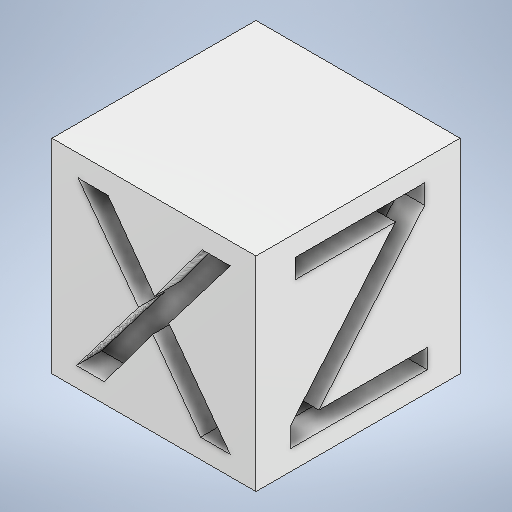
# Autodesk Inventor part: Cubo
Saved by Autodesk Inventor 2025.2 (Build 292293000, 293)
## iProperties
Created: 2025-01-18
Part Number: Cubo
Material: ABS Plastic
Document SubType Name: Modeling
Designer: Tony Dias
Density: 1.06 g/cm^3
Appearance: Smooth - White
Author: Tony Dias
## iProperties of the stored document Cubo_3DPrint.ipt
Created: 2025-01-18
Part Number: Cubo_3DPrint
Material: Generic
Document SubType Name: Modeling
Designer: Tony Dias
Density: 1 g/cm^3
Appearance: Default
Author: Tony Dias
Autodesk Inventor part; units mm, degrees
ref_plane "YZ Plane" through (0, 0, 0) normal (1, 0, 0) x (0, 1, 0)
ref_plane "XZ Plane" through (0, 0, 0) normal (0, 1, 0) x (-1, 0, 0)
ref_plane "XY Plane" through (0, 0, 0) normal (0, 0, 1) x (1, 0, 0)
sketch "Sketch3" plane through (0, 0, 0) normal (0, 0, 1) x (1, 0, 0)
  line L0 (12.7, -12.7) -> (-12.7, -12.7)
  line L1 (-12.7, -12.7) -> (-12.7, 12.7)
  line L2 (-12.7, 12.7) -> (12.7, 12.7)
  line L3 (12.7, 12.7) -> (12.7, -12.7)
  line L4 (12.7, -12.7) -> (-12.7, 12.7) construction
  line L5 (-12.7, -12.7) -> (12.7, 12.7) construction
  point P0 (0, 0)
  dimension "d0" = 25.4
  dimension "d1" = 25.4
  constraints: 12 end point, 2 midpoint, 2 parallel, 1 horizontal, 1 perpendicular
  measures "d0" distance of L1.end L2.end
  measures "d1" distance of L0.end L1.end
extrude "Cubo" add sketch "Sketch3" along normal blind 25.4
sketch "Sketch5" plane through (0, 0, 25.4) normal (0, 0, 1) x (1, 0, 0)
  line L0 (-12.1868, 12.0555) -> (12.0292, 12.0555) construction
  line L1 (12.0292, 12.0555) -> (12.0292, -12.3181) construction
  line L2 (12.0292, -12.3181) -> (-12.1868, -12.3181) construction
  line L3 (-12.1868, -12.3181) -> (-12.1868, 12.0555) construction
  line L4 (9.4966, -10.2913) -> (5.7916, -10.2913)
  line L5 (5.7916, -10.2913) -> (-0.1365, -2.1567)
  line L6 (-0.1365, -2.1567) -> (-6.1633, -10.2913)
  line L7 (-6.1633, -10.2913) -> (-9.6707, -10.2913)
  line L8 (-9.6707, -10.2913) -> (-1.9149, -0.1313)
  line L9 (-1.9149, -0.1313) -> (-9.4402, 10.0287)
  line L10 (-9.4402, 10.0287) -> (-5.7352, 10.0287)
  line L11 (-5.7352, 10.0287) -> (0.0776, 2.0588)
  line L12 (0.0776, 2.0588) -> (5.9892, 10.0287)
  line L13 (5.9892, 10.0287) -> (9.4966, 10.0287)
  line L14 (9.4966, 10.0287) -> (1.856, 0.0169)
  line L15 (1.856, 0.0169) -> (9.4966, -10.2913)
  point P0 (0, 0)
  constraints: 2 other
extrude "X" cut sketch "Sketch5" against normal blind 3.175
sketch "Sketch6" plane through (12.7, -12.7, 0) normal (1, 0, 0) x (0, 0, -1)
  line L0 (-25.0445, 24.9615) -> (-0.3507, 24.9615) construction
  line L1 (-0.3507, 24.9615) -> (-0.3507, 0.3203) construction
  line L2 (-0.3507, 0.3203) -> (-25.0445, 0.3203) construction
  line L3 (-25.0445, 0.3203) -> (-25.0445, 24.9615) construction
  line L4 (-4.069, 2.4809) -> (-21.0792, 2.4809)
  line L5 (-21.0792, 2.4809) -> (-21.0792, 5.0003)
  line L6 (-21.0792, 5.0003) -> (-8.0375, 20.3967)
  line L7 (-8.0375, 20.3967) -> (-20.4864, 20.3967)
  line L8 (-20.4864, 20.3967) -> (-20.4864, 22.8009)
  line L9 (-20.4864, 22.8009) -> (-4.3984, 22.8009)
  line L10 (-4.3984, 22.8009) -> (-4.3984, 20.3638)
  line L11 (-4.3984, 20.3638) -> (-17.5718, 4.885)
  line L12 (-17.5718, 4.885) -> (-4.069, 4.885)
  line L13 (-4.069, 4.885) -> (-4.069, 2.4809)
  point P0 (0, 12.7)
  constraints: 2 other
extrude "Z" cut sketch "Sketch6" against normal blind 3.175
sketch "Sketch7" plane through (0, 0, 0) normal (0, 0, -1) x (-1, 0, 0)
  line L0 (-12.3672, 12.2796) -> (12.4407, 12.2796) construction
  line L1 (12.4407, 12.2796) -> (12.4407, -12.4691) construction
  line L2 (12.4407, -12.4691) -> (-12.3672, -12.4691) construction
  line L3 (-12.3672, -12.4691) -> (-12.3672, 12.2796) construction
  line L4 (-1.8683, -10.2547) -> (-1.8683, -1.7055)
  line L5 (-1.8683, -1.7055) -> (-8.559, 10.0653)
  line L6 (-8.559, 10.0653) -> (-4.2379, 10.0653)
  line L7 (-4.2379, 10.0653) -> (0.0677, 2.0116)
  line L8 (0.0677, 2.0116) -> (4.2959, 10.0653)
  line L9 (4.2959, 10.0653) -> (8.555, 10.0653)
  line L10 (8.555, 10.0653) -> (1.8178, -1.7364)
  line L11 (1.8178, -1.7364) -> (1.8178, -10.2547)
  line L12 (1.8178, -10.2547) -> (-1.8683, -10.2547)
  point P0 (0, 0)
  constraints: 2 other
extrude "Y" cut sketch "Sketch7" against normal blind 3.175
body "Solid1"
